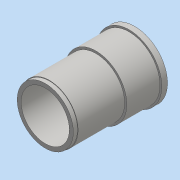
# Autodesk Inventor part: Eye-Piece
Saved by Autodesk Inventor 2016 SP1 (Build 200210100, 210)
## iProperties
Created: 2016-03-17
Part Number: Eye-Piece
Material: Generic
Document SubType Name: Modeling
Designer: Mohamed A.
Density: 1 g/cm^3
Appearance: Default
Author: Mohamed A.
Autodesk Inventor part; units mm, degrees
ref_plane "YZ Plane" through (0, 0, 0) normal (1, 0, 0) x (0, 1, 0)
ref_plane "XZ Plane" through (0, 0, 0) normal (0, 1, 0) x (-1, 0, 0)
ref_plane "XY Plane" through (0, 0, 0) normal (0, 0, 1) x (1, 0, 0)
sketch "Sketch6" plane through (0, 0, 0) normal (0, 0, 1) x (1, 0, 0)
  line L0 (11.35, 0) -> (11.35, 1.7)
  line L1 (11.35, 1.7) -> (11.6, 1.7)
  line L2 (11.6, 1.7) -> (11.6, 20.5)
  line L3 (11.6, 20.5) -> (12.5, 20.5)
  line L4 (12.5, 20.5) -> (12.5, 33.9)
  line L5 (12.5, 33.9) -> (13.25, 33.9)
  line L6 (13.25, 33.9) -> (13.25, 36.2)
  line L7 (11.35, 0) -> (9.75, 0)
  line L8 (9.75, 0) -> (9.75, 33.9)
  line L9 (13.25, 36.2) -> (5.15, 36.2)
  line L10 (5.15, 36.2) -> (5.15, 33.9)
  line L11 (5.15, 33.9) -> (9.75, 33.9)
  line L12 (0, -7.24) -> (0, 43.44) construction
  point P0 (0, 0)
  dimension "d7" = 11.35
  dimension "d8" = 1.7
  dimension "d9" = 11.6
  dimension "d11" = 12.5
  dimension "d13" = 13.25
  dimension "d14" = 2.3
  dimension "d16" = 1.6
  dimension "d17" = 8.1
  dimension "d18" = 0.25
  dimension "d19" = 15.7
  dimension "d20" = 36.2
  constraints: 24 end point, 6 perpendicular, 3 vertical, 2 horizontal, 1 collinear
  measures "d7" distance of point (0, 0) L0.start
  measures "d8" distance of L0.start L0.end
  measures "d9" horizontal distance of point (0, 0) L1.end
  measures "d11" horizontal distance of point (0, 0) L3.end
  measures "d13" horizontal distance of point (0, 0) L5.end
  measures "d14" distance of L5.end L6.end
  measures "d16" distance of L0.start L7.end
  measures "d17" distance of L6.end L9.end
  measures "d18" distance between parallel lines of L0 L2
  measures "d19" distance between parallel lines of L3 L9
  measures "d20" distance between parallel lines of L7 L9
revolve "Revolution1" add sketch "Sketch6" angle 360 about axis through (0, -10, 0) along (0, 1, 0)
body "Solid1"
